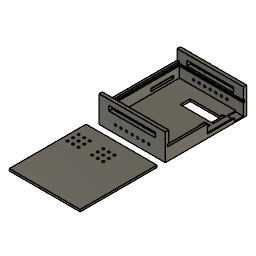
PCB_Case4v2 (Autodesk Fusion 360 design; units mm, degrees)
part number: 2026-02-18-20-16-18-437
Autodesk Fusion 360 part; units mm, degrees
note: some values were not read from the file. Set by a fixed rule: which sketch regions a step uses.
sketch "Base" plane through (0, 0, 0) normal (0, 0, 1) x (1, 0, 0)
  line L0 (29.9, 17.2774) -> (-30, 17.2774)
  line L1 (-30, 17.2774) -> (-30, -56.2226)
  line L2 (-30, -56.2226) -> (29.9, -56.2226)
  line L3 (29.9, -56.2226) -> (29.9, 17.2774)
  dimension "d3" = 59.9
  dimension "d4" = 73.5
  constraint horizontal L0
  constraint vertical L1
  constraint horizontal L2
  constraint vertical L3
  measures "d3" distance of L0.start L0.end
  measures "d4" distance of L0.start L2.end
extrude "Extrude1" add sketch "Base" along normal blind 15 makes body 1
sketch "Top" plane through (0, 0, 15) normal (0, 0, 1) x (-1, 0, 0)
  line L0 (-29.9, 56.2226) -> (-29.9, -17.2774)
  line L1 (-29.9, -17.2774) -> (30, -17.2774)
  line L2 (30, -17.2774) -> (30, 56.2226)
  line L3 (30, 56.2226) -> (-29.9, 56.2226)
sketch "Main Slot" plane through (0, 0, 15) normal (0, 0, 1) x (-1, 0, 0)
  line L0 (-27.9, 53.2226) -> (28, 53.2226)
  line L1 (28, 53.2226) -> (28, -14.2774)
  line L2 (28, -14.2774) -> (-27.9, -14.2774)
  line L3 (-27.9, -14.2774) -> (-27.9, 53.2226)
  line L4 (-29.9, 56.2226) -> (-29.9, -17.2774)
  line L5 (30, 56.2226) -> (-29.9, 56.2226)
  line L6 (-29.9, -17.2774) -> (30, -17.2774)
  dimension "d17" = 55.9
  dimension "d18" = 67.5
  dimension "d19" = 2
  dimension "d70" = 3
  constraint horizontal L0
  constraint vertical L1
  constraint horizontal L2
  constraint vertical L3
  measures "d17" distance of L0.start L0.end
  measures "d18" distance of L0.start L2.end
  measures "d19" distance of L3 L4
  measures "d70" distance of L2 L6
extrude "Extrude4" cut sketch "Main Slot" against normal blind 13 bodies 1
sketch "Port Hole" plane through (0, 0, 15) normal (0, 0, 1) x (-1, 0, 0)
  line L0 (-29.9, 18.2226) -> (-27.9, 18.2226)
  line L1 (-27.9, 18.2226) -> (-27.9, -14.2774)
  line L2 (-27.9, -14.2774) -> (-29.9, -14.2774)
  line L3 (-29.9, -14.2774) -> (-29.9, 18.2226)
  line L4 (-27.9, -14.2774) -> (-27.9, 53.2226)
  line L5 (30, 56.2226) -> (-29.9, 56.2226)
  line L6 (-29.9, -17.2774) -> (30, -17.2774)
  dimension "d23" = 32.5
  dimension "d24" = 2
  dimension "d27" = 2
  dimension "d69" = 3
  constraint horizontal L0
  constraint vertical L1
  constraint horizontal L2
  constraint vertical L3
  measures "d23" distance of L0.start L2.end
  measures "d24" distance of L0.start L0.end
  measures "d27" distance of L3 L4
  measures "d69" distance of L2 L6
extrude "Extrude5" cut sketch "Port Hole" against normal blind 11.5 bodies 1
sketch "Antenna Hole" plane through (-30, 0, 0) normal (-1, 0, 0) x (0, -1, 0)
  line L0 (-17.2774, 0) -> (56.2226, 0)
  line L1 (56.2226, 0) -> (56.2226, 15)
  line L2 (56.2226, 15) -> (-17.2774, 15)
  line L3 (-17.2774, 15) -> (-17.2774, 0)
  line L4 (-9.1774, 5.73) -> (11.3226, 5.73)
  line L5 (11.3226, 5.73) -> (11.3226, 4.23)
  line L6 (11.3226, 4.23) -> (-9.1774, 4.23)
  line L7 (-9.1774, 4.23) -> (-9.1774, 5.73)
  line L8 (-17.2774, 0) -> (56.2226, 0)
  dimension "d36" = 20.5
  dimension "d37" = 1.5
  dimension "d39" = 4.23
  dimension "d63" = 8.1
  constraint horizontal L4
  constraint vertical L5
  constraint horizontal L6
  constraint vertical L7
  measures "d36" distance of L4.start L4.end
  measures "d37" distance of L4.start L6.end
  measures "d39" distance of L6 L8
  measures "d63" distance of L3 L7
extrude "Extrude7" cut sketch "Antenna Hole" against normal blind 2 contours L4 L5 L6 L7 bodies 1
chamfer "Chamfer1" distance 1 angle 45 1 edges at (-28, -1.0726, 5.73) on bodies 1
sketch "Lid Notch" plane through (29.9, 0, 0) normal (1, 0, 0) x (0, 1, 0)
  line L0 (14.2774, 15) -> (14.2774, 3.5)
  line L1 (14.2774, 3.5) -> (-18.2226, 3.5)
  line L2 (-18.2226, 3.5) -> (-18.2226, 15)
  line L3 (-18.2226, 15) -> (-56.2226, 15)
  line L4 (-56.2226, 15) -> (-56.2226, 0)
  line L5 (-56.2226, 0) -> (17.2774, 0)
  line L6 (17.2774, 0) -> (17.2774, 15)
  line L7 (17.2774, 15) -> (14.2774, 15)
  line L8 (-54.2226, 13.5) -> (15.2774, 13.5)
  line L9 (15.2774, 13.5) -> (15.2774, 11.5)
  line L10 (15.2774, 11.5) -> (-54.2226, 11.5)
  line L11 (-54.2226, 11.5) -> (-54.2226, 13.5)
  line L12 (-133.0862, 1.91) -> (-63.6862, 1.91)
  line L13 (-63.6862, 1.91) -> (-63.6862, 0)
  line L14 (-63.6862, 0) -> (-133.0862, 0)
  line L15 (-133.0862, 0) -> (-133.0862, 1.91)
  dimension "d46" = 69.5
  dimension "d47" = 2
  dimension "d50" = 11.5
  dimension "d64" = 69.4
  dimension "d65" = 1.91
  dimension "d68" = 2
  constraint horizontal L8
  constraint vertical L9
  constraint horizontal L10
  constraint vertical L11
  constraint horizontal L12
  constraint vertical L13
  constraint horizontal L14
  constraint vertical L15
  constraint collinear L5 L14
  measures "d46" distance of L8.start L8.end
  measures "d47" distance of L8.start L10.end
  measures "d50" distance of L5 L10
  measures "d64" distance of L12.start L12.end
  measures "d65" distance of L12.end L13.end
  measures "d68" distance of L6 L9
extrude "Notch" cut sketch "Lid Notch" against normal blind 58.9 contours L0 L8 L9 L10 | L0 L2 L8 L10 | L2 L8 L10 L11 bodies 1
extrude "Lid" add sketch "Lid Notch" against normal blind 64 separate body contours L12 L13 L14 L15 makes body 2
sketch "Inductor Space" plane through (0, 0, 2) normal (0, 0, 1) x (-1, 0, 0)
  line L0 (-27.9, -14.2774) -> (28, -14.2774)
  line L1 (28, -14.2774) -> (28, 53.2226)
  line L2 (28, 53.2226) -> (-27.9, 53.2226)
  line L3 (-27.9, 53.2226) -> (-27.9, -14.2774)
  line L4 (-22.9, 13.7226) -> (-17.9, 13.7226)
  line L5 (-17.9, 13.7226) -> (-17.9, 8.7226)
  line L6 (-17.9, 8.7226) -> (-22.9, 8.7226)
  line L7 (-22.9, 8.7226) -> (-22.9, 13.7226)
  dimension "d55" = 5
  dimension "d56" = 5
  dimension "d57" = 5
  dimension "d62" = 23
  constraint horizontal L4
  constraint vertical L5
  constraint horizontal L6
  constraint vertical L7
  measures "d55" distance of L4.start L4.end
  measures "d56" distance of L4.end L5.end
  measures "d57" distance of L3 L7
  measures "d62" distance of L0 L6
extrude "Extrude11" cut sketch "Inductor Space" against normal blind 1 contours L4 L5 L6 L7 bodies 1
sketch "Bottom Sensor Hole" plane through (0, 0, 2) normal (0, 0, 1) x (-1, 0, 0)
  line L0 (-17.9, 13.7226) -> (-17.9, 8.7226)
  line L1 (-17.9, 8.7226) -> (-22.9, 8.7226)
  line L2 (-22.9, 8.7226) -> (-22.9, 13.7226)
  line L3 (-22.9, 13.7226) -> (-17.9, 13.7226)
  line L4 (-27.9, -14.2774) -> (28, -14.2774)
  line L5 (28, -14.2774) -> (28, 53.2226)
  line L6 (28, 53.2226) -> (-27.9, 53.2226)
  line L7 (-27.9, 53.2226) -> (-27.9, -14.2774)
  line L8 (-20.248, 5.9276) -> (6.752, 5.9276)
  line L9 (6.752, 5.9276) -> (6.752, -2.8724)
  line L10 (6.752, -2.8724) -> (-20.248, -2.8724)
  line L11 (-20.248, -2.8724) -> (-20.248, 5.9276)
  line L12 (-29.9, 54.2226) -> (-29.9, -15.2774)
  dimension "d73" = 27
  dimension "d74" = 8.8
  dimension "d75" = 9.652
  dimension "d76" = 11.405
  constraint horizontal L8
  constraint vertical L9
  constraint horizontal L10
  constraint vertical L11
  measures "d73" distance of L8.start L8.end
  measures "d74" distance of L8.start L10.end
  measures "d75" distance of L11 L12
  measures "d76" distance of L4 L10
extrude "Extrude14" cut sketch "Bottom Sensor Hole" against normal blind 2 contours L8 L9 L10 L11 bodies 1
sketch "Sketch14" plane through (0, 0, 15) normal (0, 0, 1) x (-1, 0, 0)
  line L0 (28, -14.2774) -> (-29.9, -14.2774)
  line L1 (-29.9, -14.2774) -> (-29.9, -17.2774)
  line L2 (-29.9, -17.2774) -> (30, -17.2774)
  line L3 (30, -17.2774) -> (30, 56.2226)
  line L4 (30, 56.2226) -> (-29.9, 56.2226)
  line L5 (-29.9, 56.2226) -> (-29.9, 18.2226)
  line L6 (-29.9, 18.2226) -> (-27.9, 18.2226)
  line L7 (-27.9, 18.2226) -> (-27.9, 53.2226)
  line L8 (-27.9, 53.2226) -> (28, 53.2226)
  line L9 (28, 53.2226) -> (28, -14.2774)
  line L10 (-29.9, 18.2226) -> (-27.9, 18.2226)
  line L11 (-27.9, 18.2226) -> (-27.9, 53.2226)
  line L12 (-27.9, 53.2226) -> (-29.9, 53.2226)
  line L13 (-29.9, 53.2226) -> (-29.9, 18.2226)
  constraint horizontal L10
  constraint vertical L11
  constraint horizontal L12
  constraint vertical L13
  constraint coincident L7.end L8.start
  constraint coincident L5.end L6.start
extrude "Extrude15" cut sketch "Sketch14" against normal blind 2.5 contours L5 L6 L7 L10 L11 L12 L13 bodies 1
sketch "Sketch17" plane through (0, -56.2226, 0) normal (0, -1, 0) x (1, 0, 0)
  line L0 (-30, 0) -> (29.9, 0)
  line L1 (29.9, 0) -> (29.9, 15)
  line L2 (29.9, 15) -> (-30, 15)
  line L3 (-30, 15) -> (-30, 0)
  line L4 (-30, 15) -> (29.9, 15)
  line L5 (29.9, 15) -> (29.9, 24)
  line L6 (29.9, 24) -> (-30, 24)
  line L7 (-30, 24) -> (-30, 15)
  line L8 (-21.05, 19.25) -> (20.95, 19.25)
  line L9 (20.95, 19.25) -> (20.95, 15)
  line L10 (20.95, 15) -> (-21.05, 15)
  line L11 (-21.05, 15) -> (-21.05, 19.25)
  dimension "d96" = 42
  dimension "d97" = 4.25
  dimension "d98" = 59.9
  dimension "d99" = 8.95
  dimension "d100" = 9
  constraint horizontal L4
  constraint vertical L5
  constraint horizontal L6
  constraint vertical L7
  constraint coincident L2.end L3.start
  constraint collinear L1 L5
  constraint horizontal L8
  constraint vertical L9
  constraint horizontal L10
  constraint vertical L11
  constraint collinear L4 L10
  measures "d96" distance of L8.start L8.end
  measures "d97" distance of L8.start L10.end
  measures "d98" distance of L5.end L6.end
  measures "d99" distance of L7 L11
  measures "d100" distance of L2.end L6.end
extrude "Extrude16" add sketch "Sketch17" against normal blind 73.5 contours L2 L4 L5 L6 L7 L8 L9 L11 bodies 1
sketch "Sketch18" plane through (29.9, 0, 0) normal (1, 0, 0) x (0, 1, 0)
  line L0 (14.2774, 15) -> (14.2774, 13.5)
  line L1 (14.2774, 13.5) -> (15.2774, 13.5)
  line L2 (15.2774, 13.5) -> (15.2774, 11.5)
  line L3 (15.2774, 11.5) -> (14.2774, 11.5)
  line L4 (14.2774, 11.5) -> (14.2774, 3.5)
  line L5 (14.2774, 3.5) -> (-18.2226, 3.5)
  line L6 (-18.2226, 3.5) -> (-18.2226, 11.5)
  line L7 (-18.2226, 11.5) -> (-54.2226, 11.5)
  line L8 (-54.2226, 11.5) -> (-54.2226, 13.5)
  line L9 (-54.2226, 13.5) -> (-53.2226, 13.5)
  line L10 (-53.2226, 13.5) -> (-53.2226, 15)
  line L11 (-53.2226, 15) -> (14.2774, 15)
  line L12 (17.2774, 0) -> (17.2774, 24)
  line L13 (17.2774, 24) -> (-56.2226, 24)
  line L14 (-56.2226, 24) -> (-56.2226, 0)
  line L15 (-56.2226, 0) -> (17.2774, 0)
  line L16 (-53.2226, 13.5) -> (14.2774, 13.5)
  line L17 (14.2774, 13.5) -> (14.2774, 24)
  line L18 (14.2774, 24) -> (-53.2226, 24)
  line L19 (-53.2226, 24) -> (-53.2226, 13.5)
  constraint horizontal L16
  constraint vertical L17
  constraint horizontal L18
  constraint vertical L19
  constraint coincident L13 L17.end
  constraint coincident L9.end L10.start
extrude "Extrude17" cut sketch "Sketch18" against normal blind 59.9 contours L11 L13 L17 L18 L19 bodies 1
sketch "Lid Holes" plane through (0, 0, 1.91) normal (0, 0, 1) x (-1, 0, 0)
  line L0 (-29.9, 133.0862) -> (-29.9, 63.6862)
  line L1 (-29.9, 63.6862) -> (34.1, 63.6862)
  line L2 (34.1, 63.6862) -> (34.1, 133.0862)
  line L3 (34.1, 133.0862) -> (-29.9, 133.0862)
  circle A0 centre (24.35, 80.1862) radius 1
  circle A1 centre (2.1, 80.1862) radius 1
  dimension "d110" = 2
  dimension "d113" = 16.5
  dimension "d114" = 9.75
  dimension "d119" = 2
  dimension "d120" = 16.5
  dimension "d121" = 32
  measures "d110" diameter of A0
  measures "d113" distance of L1 A0.centre
  measures "d114" distance of L2 A0.centre
  measures "d119" diameter of A1
  measures "d120" distance of L1 A1.centre
  measures "d121" distance of L2 A1.centre
extrude "Extrude18" cut sketch "Lid Holes" against normal blind 2 contours A0 | A1 bodies 2
pattern_linear "R-Pattern1" count 3 spacing 5 along (1, 0, 0) both ways count 3 spacing 5 along (0, -1, 0) both ways of "Extrude18"
sketch "Wall Holes" plane through (0, -56.2226, 0) normal (0, -1, 0) x (1, 0, 0)
  line L0 (20.95, 15) -> (-21.05, 15)
  line L1 (-21.05, 15) -> (-21.05, 19.25)
  line L2 (-21.05, 19.25) -> (20.95, 19.25)
  line L3 (20.95, 19.25) -> (20.95, 15)
  line L4 (29.9, 0) -> (29.9, 24)
  line L5 (29.9, 24) -> (-30, 24)
  line L6 (-30, 24) -> (-30, 0)
  line L7 (-30, 0) -> (29.9, 0)
  circle A0 centre (-0.05, 7) radius 1
  line L8 (27.9, 2) -> (-28, 2)
  line L9 (27.9, 11.5) -> (27.9, 2)
  dimension "d122" = 2
  dimension "d123" = 5
  dimension "d131" = 59.9
  dimension "d132" = 29.95
  measures "d122" diameter of A0
  measures "d123" distance of A0.centre L8
  measures "d131" distance of L4.end L5.end
  measures "d132" distance of L4 A0.centre
extrude "Extrude19" cut sketch "Wall Holes" against normal blind 73.5 contours A0 bodies 1
pattern_linear "R-Pattern2" count 7 spacing 5 along (1, 0, 0) both ways of "Extrude19"
sketch "Battery Wire Hole" plane through (27.9, 0, 0) normal (-1, 0, 0) x (0, -1, 0)
  line L0 (53.2226, 11.5) -> (18.2226, 11.5)
  line L1 (18.2226, 11.5) -> (18.2226, 3.5)
  line L2 (18.2226, 3.5) -> (-14.2774, 3.5)
  line L3 (-14.2774, 3.5) -> (-14.2774, 2)
  line L4 (-14.2774, 2) -> (53.2226, 2)
  line L5 (53.2226, 2) -> (53.2226, 11.5)
  line L6 (-14.2774, 2) -> (-6.2774, 2)
  line L7 (-6.2774, 2) -> (-6.2774, 3.5)
  line L8 (-6.2774, 3.5) -> (-14.2774, 3.5)
  line L9 (-14.2774, 3.5) -> (-14.2774, 2)
  dimension "d133" = 1.5
  dimension "d134" = 8
  constraint horizontal L6
  constraint vertical L7
  constraint horizontal L8
  constraint vertical L9
  constraint coincident L2 L7.end
  constraint coincident L3.end L4.start
  measures "d133" distance of L6.end L7.end
  measures "d134" distance of L7.end L2.end
extrude "Extrude20" cut sketch "Battery Wire Hole" against normal blind 2 contours L2 L3 L4 L6 L7 L8 L9 bodies 1
sketch "Sketch22" plane through (0, 0, 3.5) normal (0, 0, 1) x (-1, 0, 0)
  line L0 (-29.9, -6.2774) -> (-27.9, -6.2774)
  line L1 (-27.9, -6.2774) -> (-27.9, 18.2226)
  line L2 (-27.9, 18.2226) -> (-29.9, 18.2226)
  line L3 (-29.9, 18.2226) -> (-29.9, -6.2774)
  line L4 (-27.9, -6.2774) -> (-28.9, -6.2774)
  line L5 (-28.9, -6.2774) -> (-28.9, 18.2226)
  line L6 (-28.9, 18.2226) -> (-27.9, 18.2226)
  line L7 (-27.9, 18.2226) -> (-27.9, -6.2774)
  constraint horizontal L4
  constraint vertical L5
  constraint horizontal L6
  constraint vertical L7
  constraint midpoint L2 L5.end
  constraint coincident L0.end L1.start
extrude "Extrude21" cut sketch "Sketch22" against normal blind 1.5 contours L0 L1 L2 L4 L5 L6 L7 bodies 1
sketch "Sketch23" plane through (0, 0, 2) normal (0, 0, 1) x (-1, 0, 0)
  line L0 (6.752, 5.9276) -> (6.752, -2.8724)
  line L1 (6.752, -2.8724) -> (-20.248, -2.8724)
  line L2 (-20.248, -2.8724) -> (-20.248, 5.9276)
  line L3 (-20.248, 5.9276) -> (6.752, 5.9276)
  line L4 (-17.9, 13.7226) -> (-17.9, 8.7226)
  line L5 (-17.9, 8.7226) -> (-22.9, 8.7226)
  line L6 (-22.9, 8.7226) -> (-22.9, 13.7226)
  line L7 (-22.9, 13.7226) -> (-17.9, 13.7226)
  line L8 (-29.9, -14.2774) -> (28, -14.2774)
  line L9 (28, -14.2774) -> (28, 53.2226)
  line L10 (28, 53.2226) -> (-27.9, 53.2226)
  line L11 (-27.9, 53.2226) -> (-27.9, 18.2226)
  line L12 (-28.9, -6.2774) -> (-29.9, -6.2774)
  line L13 (-29.9, -6.2774) -> (-29.9, -14.2774)
  line L14 (-29.9, -14.2774) -> (-22.9, -14.2774)
  line L15 (-22.9, -14.2774) -> (-22.9, -6.2774)
  line L16 (-22.9, -6.2774) -> (-29.9, -6.2774)
  line L17 (-29.9, -6.2774) -> (-29.9, -14.2774)
  line L18 (-27.9, 18.2226) -> (-28.9, 18.2226)
  line L19 (-28.9, 18.2226) -> (-28.9, -6.2774)
  dimension "d146" = 7
  constraint horizontal L14
  constraint vertical L15
  constraint horizontal L16
  constraint vertical L17
  constraint coincident L8.start L13.end
  constraint collinear L12 L16
  measures "d146" distance of L15.end L12.end
extrude "Extrude22" cut sketch "Sketch23" against normal blind 1 contours L8 L12 L13 L14 L15 L16 L17 bodies 1
sketch "Sketch24" plane through (0, 0, 2) normal (0, 0, 1) x (-1, 0, 0)
  line L0 (-22.9, -6.2774) -> (-22.9, -14.2774)
  line L1 (-22.9, -14.2774) -> (28, -14.2774)
  line L2 (28, -14.2774) -> (28, 53.2226)
  line L3 (28, 53.2226) -> (-27.9, 53.2226)
  line L4 (-27.9, 53.2226) -> (-27.9, 18.2226)
  line L5 (-28.9, -6.2774) -> (-22.9, -6.2774)
  line L6 (6.752, 5.9276) -> (6.752, -2.8724)
  line L7 (6.752, -2.8724) -> (-20.248, -2.8724)
  line L8 (-20.248, -2.8724) -> (-20.248, 5.9276)
  line L9 (-20.248, 5.9276) -> (6.752, 5.9276)
  line L10 (-17.9, 13.7226) -> (-17.9, 8.7226)
  line L11 (-17.9, 8.7226) -> (-22.9, 8.7226)
  line L12 (-22.9, 8.7226) -> (-22.9, 13.7226)
  line L13 (-22.9, 13.7226) -> (-17.9, 13.7226)
  line L14 (-22.9, -5.0724) -> (-19.9, -5.0724)
  line L15 (-19.9, -5.0724) -> (-19.9, 5.9276)
  line L16 (-19.9, 5.9276) -> (-22.9, 5.9276)
  line L17 (-22.9, 5.9276) -> (-22.9, -5.0724)
  line L18 (-27.9, 18.2226) -> (-28.9, 18.2226)
  line L19 (-28.9, 18.2226) -> (-28.9, -6.2774)
  dimension "d149" = 11
  dimension "d150" = 3
  constraint horizontal L14
  constraint vertical L15
  constraint horizontal L16
  constraint vertical L17
  constraint collinear L9 L16
  measures "d149" distance of L14.end L15.end
  measures "d150" distance of L14.start L14.end
extrude "Extrude23" cut sketch "Sketch24" against normal blind 1 contours L7 L8 L14 L15 L16 L17 bodies 1
extrude "Extrude2" [suppressed]
extrude "Extrude3" [suppressed]
equation "d4 = 36.5 mm + 3.7 cm"
equation "d18 = 30.5 mm + 3.7 cm"
equation "d39 = 4.48 mm - 0.25 mm"
equation "d46 = 32.5 mm + 3.7 cm"
equation "d64 = 32.5 mm - 0.1 mm + 3.7 cm"
equation "d101 = -36.5 mm - 3.7 cm"
equation "d125 = -36.5 mm - 3.7 cm"
